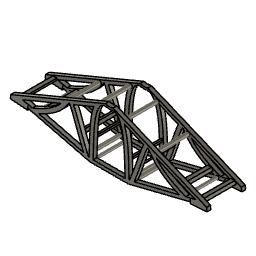
michael v2.1 (Autodesk Fusion 360 design; units mm, degrees)
Autodesk Fusion 360 part; units mm, degrees
note: some values were not read from the file. Chosen so that the rebuilt part matches the saved one: which bodies a step acts on; which face or edge a step refers to. Set by a fixed rule: which sketch regions a step uses.
sketch "Sketch1" plane through (0, 0, 0) normal (0, 1, 0) x (1, 0, 0)
  line L0 (25, 0) -> (1, -10)
  line L1 (1, -10) -> (-1, -10)
  line L2 (-1, -10) -> (-25, 0)
  line L3 (-25, 0) -> (-5, 5)
  line L4 (-5, 5) -> (5, 5)
  line L5 (5, 5) -> (25, 0)
  spline S0 degree 5 poles (-20, 1) (-19.2403, 0.7047) (-17.8035, 0.1022) (-15.8964, -0.8381) (-13.849, -2.1619) (-12.0856, -3.8766) (-10.9993, -5.4228) (-10.3856, -6.4426) (-9.8161, -6.1225) (-8.8356, -3.7469) (-7.5436, -0.1377) (-6.2085, 3.4206) (-5.1734, 5.4988) (-4.6658, 5.0904) (-4.5881, 2.2267) (-4.557, -2.0543) (-4.1341, -6.3381) (-3.0776, -9.3259) (-1.4192, -10.3031) (0.0018, -9.8007) (0.0297, -9.8291) (1.5281, -10.3066) (3.1476, -9.1997) (4.1871, -6.1078) (4.5919, -1.7775) (4.6236, 2.4585) (4.7028, 5.1964) (5.2006, 5.4318) (6.1954, 3.2085) (7.4642, -0.4237) (8.6808, -4.0195) (9.5989, -6.3084) (10.1455, -6.5191) (10.7877, -5.4507) (11.919, -3.8715) (13.7372, -2.1454) (15.8293, -0.8218) (17.7701, 0.1124) (19.2292, 0.7086) (20, 1) knots 0 0 0 0 0 0 0.028571 0.057143 0.085714 0.114286 0.142857 0.171429 0.2 0.228571 0.257143 0.285714 0.314286 0.342857 0.371429 0.4 0.428571 0.457143 0.485714 0.514286 0.542857 0.571429 0.6 0.628571 0.657143 0.685714 0.714286 0.742857 0.771429 0.8 0.828571 0.857143 0.885714 0.914286 0.942857 0.971429 1 1 1 1 1 1
  line L6 (-3, -10) -> (1, -10)
  line L7 (-1, -10) -> (3, -10)
  line L8 (9.0232, -6.2479) -> (10.9869, -6.2479)
  line L9 (-11.2683, -6.1382) -> (-9.2683, -6.1382)
  spline S1 degree 3 poles (-20.1769, 0.5448) (-17.2123, -0.6075) (-15.0567, -1.8867) (-13.622, -3.1606) (-12.8434, -3.852) (-12.2718, -4.5345) (-11.8369, -5.1221) (-11.564, -5.4908) (-11.349, -5.8193) (-11.1311, -6.0904) (-10.9757, -6.2836) (-10.8281, -6.4698) (-10.5425, -6.5763) (-10.3344, -6.6538) (-10.0453, -6.6231) (-9.8529, -6.5067) (-9.5146, -6.3022) (-9.3456, -5.9885) (-9.1217, -5.5455) (-8.7264, -4.7631) (-8.2508, -3.5013) (-7.714, -2.0502) (-7.1742, -0.591) (-6.5841, 1.034) (-6.0619, 2.3143) (-5.764, 3.0447) (-5.4872, 3.6628) (-5.2638, 4.0714) (-5.2465, 4.1029) (-5.2298, 4.133) (-5.2131, 4.1622) knots 0 0 0 0 0.067718 0.067718 0.067718 0.104471 0.104471 0.104471 0.127531 0.127531 0.127531 0.143975 0.143975 0.143975 0.155952 0.155952 0.155952 0.177002 0.177002 0.177002 0.214181 0.214181 0.214181 0.251568 0.251568 0.251568 0.272898 0.272898 0.272898 0.274544 0.274544 0.274544 0.274544
  spline S2 degree 3 poles (-5.2131, 4.1622) (-5.208, 4.1249) (-5.2033, 4.0866) (-5.1986, 4.0462) (-5.0527, 2.7868) (-5.1114, -0.0655) (-4.8975, -2.8177) (-4.7462, -4.7642) (-4.4511, -6.6318) (-3.9155, -7.982) (-3.4788, -9.0829) (-2.8567, -9.8535) (-2.1561, -10.2132) (-1.4917, -10.5542) (-0.8223, -10.5033) (-0.4331, -10.4359) (-0.1843, -10.3928) (-0.0637, -10.364) (-0.0009, -10.3634) (0.0638, -10.3627) (0.1714, -10.3893) (0.4222, -10.4337) (0.8186, -10.5039) (1.526, -10.5596) (2.2152, -10.1811) (2.9971, -9.7517) (3.6572, -8.8068) (4.1011, -7.4721) (4.6761, -5.743) (4.9244, -3.3252) (5.0281, -1.0519) (5.0946, 0.4047) (5.1084, 1.7848) (5.1461, 2.83) (5.1636, 3.3151) (5.1866, 3.7296) (5.2195, 4.045) knots 0.318472 0.318472 0.318472 0.318472 0.320269 0.320269 0.320269 0.376395 0.376395 0.376395 0.41609 0.41609 0.41609 0.448454 0.448454 0.448454 0.479141 0.479141 0.479141 0.498761 0.498761 0.498761 0.518936 0.518936 0.518936 0.550826 0.550826 0.550826 0.587009 0.587009 0.587009 0.633885 0.633885 0.633885 0.663919 0.663919 0.663919 0.677857 0.677857 0.677857 0.677857
  spline S3 degree 3 poles (5.2195, 4.045) (5.7787, 2.9299) (6.6595, 0.3726) (7.4382, -1.8648) (7.8608, -3.0791) (8.2541, -4.1927) (8.5917, -5.0079) (8.8482, -5.6274) (9.0535, -6.067) (9.3196, -6.3771) (9.4638, -6.5451) (9.6592, -6.702) (9.921, -6.7316) (10.1799, -6.7608) (10.4059, -6.6441) (10.5551, -6.5239) (10.8591, -6.2791) (11.0478, -5.9647) (11.3162, -5.5889) (11.9413, -4.7139) (12.8726, -3.5471) (14.392, -2.4312) (15.8105, -1.3894) (17.7282, -0.3811) (20.1727, 0.5432) knots 0.725805 0.725805 0.725805 0.725805 0.78204 0.78204 0.78204 0.812559 0.812559 0.812559 0.835746 0.835746 0.835746 0.848309 0.848309 0.848309 0.860733 0.860733 0.860733 0.88604 0.88604 0.88604 0.944978 0.944978 0.944978 1 1 1 1
  line L10 (-1.3166, -10.7599) -> (-27.6104, 0.1959)
  line L11 (-27.6104, 0.1959) -> (-5.1013, 5.8232)
  line L12 (-5.1013, 5.8232) -> (5.1013, 5.8232)
  line L13 (5.1013, 5.8232) -> (27.6104, 0.1959)
  line L14 (27.6104, 0.1959) -> (1.3166, -10.7599)
  line L15 (-0.6783, -9.2279) -> (-22.3474, -0.1991)
  line L16 (-22.3474, -0.1991) -> (-4.897, 4.1635)
  line L17 (-4.897, 4.1635) -> (4.897, 4.1635)
  line L18 (4.897, 4.1635) -> (22.3474, -0.1991)
  line L19 (22.3474, -0.1991) -> (0.6783, -9.2279)
  spline S4 degree 3 poles (-19.7998, 1.5152) (-16.8225, 0.3581) (-14.5773, -0.9467) (-13.0307, -2.2941) (-12.167, -3.0467) (-11.5203, -3.8057) (-11.045, -4.4423) (-10.7165, -4.8822) (-10.4611, -5.2685) (-10.2922, -5.4716) (-10.2892, -5.4752) (-10.2863, -5.4787) (-10.2834, -5.4822) knots 0 0 0 0 0.066275 0.066275 0.066275 0.10329 0.10329 0.10329 0.128875 0.128875 0.128875 0.129325 0.129325 0.129325 0.129325
  spline S5 degree 3 poles (-10.2834, -5.4822) (-10.213, -5.3798) (-10.1216, -5.2198) (-10.0196, -5.0131) (-9.5021, -3.9637) (-8.6841, -1.6464) (-7.8582, 0.56) (-7.285, 2.0914) (-6.7235, 3.5271) (-6.2535, 4.4282) (-6.0622, 4.7949) (-5.9002, 5.0727) (-5.6759, 5.2944) (-5.5547, 5.4142) (-5.399, 5.547) (-5.1337, 5.5697) (-4.9199, 5.588) (-4.6829, 5.4776) (-4.5586, 5.35) (-4.3362, 5.1218) (-4.2946, 4.9035) (-4.24, 4.6478) (-4.1128, 4.051) (-4.0809, 3.1735) (-4.051, 2.0524) (-3.9922, -0.1505) (-3.9424, -3.2017) (-3.5166, -5.5027) (-3.2569, -6.9057) (-2.8534, -8.0081) (-2.4018, -8.6306) (-1.8296, -9.4191) (-1.2594, -9.4836) (-0.8004, -9.4366) (-0.5153, -9.4074) (-0.2866, -9.3198) (0.0148, -9.3222) (0.3745, -9.3251) (0.6299, -9.4457) (0.9926, -9.4472) (1.4364, -9.4491) (1.9561, -9.2967) (2.4738, -8.5216) (2.9611, -7.7919) (3.379, -6.4966) (3.6305, -4.9034) (4.0351, -2.3397) (4.0309, 0.9103) (4.1091, 2.9608) (4.1384, 3.7298) (4.1753, 4.3202) (4.2787, 4.7583) (4.3253, 4.9559) (4.367, 5.1309) (4.5365, 5.3242) (4.6434, 5.4461) (4.8535, 5.5715) (5.0687, 5.5696) (5.3432, 5.5671) (5.5088, 5.43) (5.6246, 5.3165) (5.8653, 5.0807) (6.0159, 4.7915) (6.2072, 4.3958) (6.7056, 3.3652) (7.3239, 1.6308) (7.939, -0.1343) (8.4375, -1.5647) (8.9236, -2.9894) (9.3243, -4.0326) (9.6013, -4.7537) (9.8455, -5.297) (10.0097, -5.5587) (10.0151, -5.5674) (10.0205, -5.5757) (10.0257, -5.5837) knots 0.16734312 0.16734312 0.16734312 0.16734312 0.17812314 0.17812314 0.17812314 0.23284777 0.23284777 0.23284777 0.27082954 0.27082954 0.27082954 0.28628713 0.28628713 0.28628713 0.29464228 0.29464228 0.29464228 0.30137353 0.30137353 0.30137353 0.31341352 0.31341352 0.31341352 0.34150932 0.34150932 0.34150932 0.39671741 0.39671741 0.39671741 0.43038234 0.43038234 0.43038234 0.47302917 0.47302917 0.47302917 0.49951678 0.49951678 0.49951678 0.5311271 0.5311271 0.5311271 0.56980573 0.56980573 0.56980573 0.60621464 0.60621464 0.60621464 0.66480001 0.66480001 0.66480001 0.68676953 0.68676953 0.68676953 0.69667909 0.69667909 0.69667909 0.70292706 0.70292706 0.70292706 0.7108975 0.7108975 0.7108975 0.72746295 0.72746295 0.72746295 0.77061347 0.77061347 0.77061347 0.8055848 0.8055848 0.8055848 0.82975991 0.82975991 0.82975991 0.83055942 0.83055942 0.83055942 0.83055942
  spline S6 degree 3 poles (10.0257, -5.5837) (10.0968, -5.4989) (10.1852, -5.38) (10.2862, -5.2397) (10.7376, -4.6118) (11.4447, -3.6101) (12.5098, -2.6306) (13.9838, -1.2749) (16.152, 0.0591) (19.0565, 1.2256) (19.3007, 1.3237) (19.55, 1.4208) (19.8045, 1.517) knots 0.869276 0.869276 0.869276 0.869276 0.880006 0.880006 0.880006 0.927997 0.927997 0.927997 0.994416 0.994416 0.994416 1 1 1 1
  point P0 (-10.2683, -6.1382)
  point P1 (10.005, -6.2479)
  dimension "d1" = 0.4884
  dimension "d2" = -0.8232
  dimension "d3" = 0.8365
  dimension "d4" = -0.5528
  constraint midpoint L1.end L6
  constraint midpoint L0.end L7
  constraint coincident L1.end L2.start
  constraint coincident L0.end L1.start
  constraint parallel L1 L6
  constraint midpoint P1 L8
  constraint midpoint P0 L9
sketch "Sketch2" plane through (0, 0, 0) normal (0, 1, 0) x (1, 0, 0)
extrude "Extrude1" add sketch "Sketch1" against normal blind 1 contours L0 L5 S3 L18 L19 S6 | L0 S0 S3 L19 | L5 L18 S5 S6 | L0 S0 L19 S5 S6 | S0 S3 L18 L19 | L5 S0 L18 S5 | S0 L18 L19 S6 | S0 L8 S3 L19 | L0 L8 S3 | L0 S2 S3 L19 | L5 S0 L17 L18 | L4 L17 S5 | L4 S0 L17 S5 | S0 L18 L19 S5 | S0 S2 S3 L17 L18 L19 | L0 S0 S2 L19 | L4 S0 L17 S5 | S0 L17 L19 S5 | L0 L2 S0 L15 L19 S5 | L3 S0 S1 S2 L16 L17 | L3 L16 S4 S5 | L3 S0 L16 S5 | S0 L15 L17 S5 | S0 S2 L15 L16 L17 | L2 L3 S1 L15 L16 S4 | S0 L15 L16 S5 | L2 S0 S2 L15 | L2 S1 S2 L15 | S0 S1 L15 L16 | S0 L15 L16 S4 | L2 S0 L15 S4 S5 | L2 L9 S1 | S0 L9 S1 L15 | L2 S0 S1 L15 | S0 S1 L15 L16 picked at (9.5826, -6.3701) picked at (-9.8509, -6.2762) makes body 1
sketch "Sketch3" plane through (0, 0, 0) normal (0, 1, 0) x (1, 0, 0)
  line L0 (22.5, -0.5) -> (23.5, -0.5)
  line L1 (23.5, -0.5) -> (24, 0)
  line L2 (24, 0) -> (22.5, 0)
  line L3 (22.5, 0) -> (22.5, -0.5)
  line L4 (-22.5, -0.5) -> (-23.5, -0.5)
  line L5 (-23.5, -0.5) -> (-24, 0)
  line L6 (-24, 0) -> (-22.5, 0)
  line L7 (-22.5, 0) -> (-22.5, -0.5)
  line L8 (-18, 0) -> (-17.5, -0.5)
  line L9 (-17.5, -0.5) -> (-16.5, -0.5)
  line L10 (-16.5, -0.5) -> (-17, 0)
  line L11 (-17, 0) -> (-18, 0)
  line L12 (17.5, -0.5) -> (18, 0)
  line L13 (18, 0) -> (17, 0)
  line L14 (17, 0) -> (16.5, -0.5)
  line L15 (16.5, -0.5) -> (17.5, -0.5)
  line L16 (8, -0.5) -> (7.5, 0)
  line L17 (7.5, 0) -> (7, 0)
  line L18 (7, 0) -> (7.5, -0.5)
  line L19 (7.5, -0.5) -> (8, -0.5)
  line L20 (4.5, 0) -> (4.5, -0.5)
  line L21 (4.5, -0.5) -> (5, -0.5)
  line L22 (5, -0.5) -> (5, 0)
  line L23 (5, 0) -> (-4.5, -0.5)
  line L24 (-4.5, -0.5) -> (-4.5, 0)
  line L25 (-4.5, 0) -> (-5, 0)
  line L26 (-5, 0) -> (-5, -0.5)
  line L27 (-5, -0.5) -> (-4.5, -0.5)
  line L28 (-8, -0.5) -> (-7.5, 0)
  line L29 (-7.5, 0) -> (-7, 0)
  line L30 (-7, 0) -> (-7.5, -0.5)
  line L31 (-7.5, -0.5) -> (-8, -0.5)
  circle A0 centre (3.5, -8.3) radius 0.5
  circle A1 centre (-3.5, -8.3) radius 0.5
  circle A2 centre (11.5, -5) radius 0.5
  circle A3 centre (-11.5, -5) radius 0.5
  circle A4 centre (-9.5, -6) radius 0.3
  circle A5 centre (9.5, -6) radius 0.3
  circle A6 centre (6, 4) radius 0.5
  circle A7 centre (-6, 4) radius 0.5
  circle A8 centre (-4.5, 4.5) radius 0.4
  circle A9 centre (4.5, 4.5) radius 0.4
  circle A10 centre (-19, 1) radius 0.4
  circle A11 centre (19, 1) radius 0.4
  constraint horizontal L0
  constraint parallel L0 L2
  constraint perpendicular L2 L3
  constraint perpendicular L3 L4
  constraint perpendicular L1 L5
  constraint parallel L4 L6
  constraint perpendicular L4 L7
  constraint horizontal L9
  constraint parallel L8 L10
  constraint parallel L9 L11
  constraint perpendicular L10 L12
  constraint parallel L9 L13
  constraint perpendicular L10 L14
  constraint parallel L9 L15
  constraint horizontal L17
  constraint parallel L16 L18
  constraint parallel L17 L19
  constraint vertical L20
  constraint perpendicular L20 L21
  constraint perpendicular L21 L22
  constraint perpendicular L21 L24
  constraint perpendicular L24 L25
  constraint perpendicular L21 L26
  constraint perpendicular L24 L27
  constraint perpendicular L26 L29
  constraint parallel L28 L30
  constraint parallel L29 L31
extrude "Extrude2" add sketch "Sketch3" along normal blind 4 contours L0 L1 L2 L3 | L4 L5 L6 L7 | L8 L9 L10 L11 | L12 L13 L14 L15 | L16 L17 L18 L19 | L20 L21 L22 L23 | L24 L25 L26 L27 | L28 L29 L30 L31 | A0 | A1 | A2 | A3 | A6 | A7 | A8 | A9 | A10 | A11 bodies 1
ref_plane "WorkPlane1" through (4.75, 4, 0.25) normal (0, 1, 0) x (0, 0, 1)
mirror "Mirror1" about plane through (4.75, 4, 0.25) normal (0, 1, 0) of bodies 1 merged
ref_plane "WorkPlane2" through (21, 0, 0) normal (1, 0, 0) x (0, 1, 0)
ref_plane "WorkPlane3" through (-21, 0, 0) normal (1, 0, 0) x (0, 1, 0)
split "Split1" by plane through (21, 0, 0) normal (1, 0, 0) bodies 1 makes body 2 at (23.5, 1.3333, 0)
split "Split2" by plane through (-21, 0, 0) normal (1, 0, 0) bodies 1 makes body 3 at (10.5089, -0.3333, -3.6228)
move_face "MoveFace1" to x (0.984808, 0, -0.173648) y (0, 1, 0) z (0.173648, 0, 0.984808) at (0.3994, 0, 4.2183) 2 faces at (22.3333, -0.3333, -0.6667) (22.3333, 8.3333, -0.6667) on bodies 2
move_face "MoveFace2" to x (0.984808, 0, 0.173648) y (0, 1, 0) z (-0.173648, 0, 0.984808) at (-0.4138, 0, 4.1274) 2 faces at (-23.6667, -0.3333, -0.3333) (-23.6667, 8.3333, -0.3333) on bodies 1
extrude "Extrude3" add 2 faces at (-23.9625, -0.3333, -0.2894) (-23.9625, 8.3333, -0.2894) along direction (-0.070387, 0, -0.99752) blind 1 on bodies 1 bodies 1 3
extrude "Extrude4" add 2 faces at (23.8367, -0.6667, -0.2064) (23.8367, 8.6667, -0.2064) along direction (0.070387, 0, -0.99752) blind 1 on bodies 2 bodies 2 1
scale "Scale1" factor 1.89274 about (-1, 8, 10) bodies 2
scale "Scale2" factor 3.07793 about (2.7855, 8, 10) bodies 2
